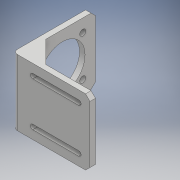
# Autodesk Inventor part: mount
Saved by Autodesk Inventor 2018 (Build 220112000, 112)
## iProperties
Created: 2018-04-10
Part Number: mount
Material: Generic
Document SubType Name: Modeling
Designer: m234547
Density: 1 g/cm^3
Appearance: Default
Author: m234547
Autodesk Inventor part; units mm, degrees
ref_plane "YZ Plane" through (0, 0, 0) normal (1, 0, 0) x (0, 1, 0)
ref_plane "XZ Plane" through (0, 0, 0) normal (0, 1, 0) x (-1, 0, 0)
ref_plane "XY Plane" through (0, 0, 0) normal (0, 0, 1) x (1, 0, 0)
sketch "Sketch5" plane through (0, 0, 0) normal (1, 0, 0) x (0, 1, 0)
  line L0 (30, 30) -> (30, -30)
  line L1 (30, -30) -> (-35, -30)
  line L2 (-35, -30) -> (-35, 30)
  line L3 (30, 30) -> (-35, 30)
  circle A0 centre (0, 0) radius 20.5
  circle A1 centre (18.385, 18.385) radius 2.75
  circle A2 centre (18.385, -18.385) radius 2.75
  circle A3 centre (-18.385, 18.385) radius 2.75
  circle A4 centre (-18.385, -18.385) radius 2.75
  dimension "d47" = 60
  dimension "d48" = 65
  dimension "d49" = 60
  dimension "d50" = 41
  dimension "d55" = 5.5
  dimension "d56" = 5.5
  dimension "d57" = 5.5
  dimension "d58" = 5.5
  constraints: 8 end point, 5 centre point, 2 perpendicular, 1 coincident, 1 vertical
  measures "d47" distance of L0.start L0.end
  measures "d48" distance of L0.end L1.end
  measures "d49" distance of L1.end L2.end
  measures "d50" diameter of A0
  measures "d55" diameter of A1
  measures "d56" diameter of A2
  measures "d57" diameter of A3
  measures "d58" diameter of A4
extrude "Extrusion5" add sketch "Sketch5" along normal blind 5
sketch "Sketch6" plane through (0, -35, -30) normal (0, -1, 0) x (1, 0, 0)
  line L0 (0, 60) -> (0, 0) projected
  line L1 (0, 60) -> (70, 60)
  line L2 (70, 60) -> (70, 0)
  line L3 (70, 0) -> (0, 0)
  line L4 (0, 0) -> (0, 60)
  line L5 (70, 60) -> (59.8, 60)
  arc A0 (59.8, 47.85) -> (59.8, 52.15) centre (59.8, 50) ccw
  arc A1 (59.8, 7.85) -> (59.8, 12.15) centre (59.8, 10) ccw
  arc A2 (18.1, 52.15) -> (18.1, 47.85) centre (18.1, 50) ccw
  arc A3 (18.1, 12.15) -> (18.1, 7.85) centre (18.1, 10) ccw
  line L6 (59.8, 47.85) -> (18.1, 47.85)
  line L7 (59.8, 52.15) -> (18.1, 52.15)
  line L8 (59.8, 7.85) -> (18.1, 7.85)
  line L9 (59.8, 12.15) -> (18.1, 12.15)
  point P0 (0, 30)
  dimension "d61" = 70
  dimension "d62" = 60
  dimension "d65" = 4.3
  dimension "d67" = 4.3
  dimension "d69" = 4.3
  dimension "d71" = 4.3
  constraints: 18 end point, 8 point on circle, 4 centre point, 3 horizontal, 1 perpendicular, 1 point on line
  measures "d61" distance of L0.start L1.end
  measures "d62" distance of L1.end L2.end
  measures "d65" diameter of A0
  measures "d67" diameter of A1
  measures "d69" diameter of A2
  measures "d71" diameter of A3
extrude "Extrusion6" add sketch "Sketch6" along normal blind 5
chamfer "Chamfer1" distance 4 angle 45 1 edges at (2.5, 30, -30)
chamfer "Chamfer2" distance 4 angle 45 1 edges at (2.5, 30, 30)
chamfer "Chamfer3" distance 4 angle 45 1 edges at (70, -37.5, 30)
chamfer "Chamfer4" distance 4 angle 45 1 edges at (70, -37.5, -30)
fillet "Fillet2" radius 4 1 edges at (0, -40, 0)
sketch "Sketch7" plane through (0, 26, 30) normal (0, 0, 1) x (1, 0, 0)
  line L0 (5, -61) -> (66, -61) projected
  line L1 (5, -61) -> (25, -61)
  line L2 (5, -61) -> (5, -41)
  line L3 (5, -61) -> (5, 0) projected
  line L4 (5, -41) -> (25, -61)
  point P0 (0, -26)
  dimension "d87" = 20
  dimension "d88" = 20
  constraints: 6 end point, 2 point on line
  measures "d87" distance of L0.start L1.end
  measures "d88" distance of L0.start L2.end
extrude "Extrusion7" add sketch "Sketch7" against normal blind 3
sketch "Sketch8" plane through (5, 26, -30) normal (0, 0, -1) x (-1, 0, 0)
  line L0 (0, -61) -> (-61, -61) projected
  line L1 (0, 0) -> (0, -41) projected
  line L2 (0, -61) -> (0, -41)
  line L3 (-20, -61) -> (0, -41) projected
  line L4 (0, -61) -> (-20, -61)
  line L5 (-20, -61) -> (0, -41)
  point P0 (5, -26)
  constraints: 6 end point, 1 collinear, 1 horizontal, 1 vertical
extrude "Extrusion8" add sketch "Sketch8" against normal blind 3
body "Solid2"
